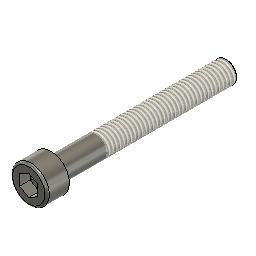
In-tube Belt Clamp (Autodesk Fusion 360 archive; units mm, degrees)
design "Hexagon Socket Head Cap Screw ANSI B18.3 - 10-32 UNF x 1 1/2 Steel Grade 2 Plain"
description: Hexagon Socket Head Cap Screw ANSI B18.3 - 10-32 UNF x 1 1/2
part number: HSHCS ANSI B18.3 - 10-32 UNF x 1 1/2 Steel Grade 2 Plain
Autodesk Fusion 360 part; units mm, degrees
sketch "Sketch1" plane through (0, 0, 0) normal (0, 1, 0) x (1, 0, 0)
  line L0 (-2.413, 0) -> (-2.413, 38.1)
  line L1 (-2.413, 38.1) -> (0, 38.1)
  line L2 (0, 38.1) -> (0, -4.826)
  line L3 (-2.413, 0) -> (-3.9624, 0)
  line L4 (-3.9624, 0) -> (-3.9624, -4.826)
  line L5 (-3.9624, -4.826) -> (0, -4.826)
  dimension "d107" = 4.826
  dimension "d108" = 38.1
  dimension "d114" = 7.9248
  dimension "d115" = 4.826
  constraint perpendicular L0 L1
  constraint collinear origin L1.end L2.end
  constraint perpendicular L0 L3
  constraint coincident origin L3
  constraint vertical L2
  constraint coincident L2 L5.end
  constraint perpendicular L2 L5
  measures "d107" distance of L3.end L5
  measures "d108" distance of origin L1
revolve "Revolve1" add sketch "Sketch1" angle 360 about axis through (0, 0, -38.1) along (0, 0, 1)
ref_plane "WorkPlane1" through (0, 0, 4.826) normal (0, 0, 1) x (1, 0, 0)
sketch "Sketch6" plane through (0, 0, 4.826) normal (0, 0, 1) x (1, 0, 0)
  line L0 (-1.9812, 1.1438) -> (-1.9812, -1.1438)
  line L1 (-1.9812, -1.1438) -> (0, -2.2877)
  line L2 (0, -2.2877) -> (1.9812, -1.1438)
  line L3 (1.9812, -1.1438) -> (1.9812, 1.1438)
  line L4 (1.9812, 1.1438) -> (0, 2.2877)
  line L5 (0, 2.2877) -> (-1.9812, 1.1438)
  dimension "d116" = 3.9624
  constraint vertical L3
  measures "d116" distance of L0 L3
extrude "Extrude1" cut sketch "Sketch6" against normal blind 2.286
extrude "Extrude2" cut 1 faces at (-0.6604, 0.3813, 2.54) along direction (0, 0, -1) blind 2.286 draft -85
thread "Thread3" "ANSI Unified Screw Threads 0.19(#10) 10-32 UNF 10-32 UNF 2A" major diameter 4.7269 minor diameter 3.8583 pitch 0.7937 angle 60 resizes the face on face at (-2.401, 0.2403, -25.4) from (0, 0, -9.652) to (0, 0, -38.1)
fillet "Fillet4" radius 0.4826 1 edges at (-3.6943, 1.4329, 4.826)
sketch "Sketch7" plane through (0, 0, 0) normal (0, 1, 0) x (1, 0, 0)
  line L0 (-2.4613, 38.1) -> (-2.4613, 37.6276)
  line L1 (-2.4613, 37.6276) -> (-1.9406, 38.1)
  line L2 (0, 38.1) -> (0, -4.826)
  line L3 (-2.4613, 38.1) -> (0, 38.1)
  dimension "d103" = 2.4613
  dimension "d110" = 1.9406
  dimension "d111" = 0.4724
  constraint coincident L2.start L3.end
  constraint perpendicular L2 L3
  constraint coincident L1.end L3
  constraint perpendicular L0 L3
  measures "d103" distance of origin L0
  measures "d110" distance of L1.end L2
  measures "d111" distance of L0.end L3
revolve "Revolve3" cut sketch "Sketch7" angle 360 about axis through (0, 0, 1.75) along (0, 0, 1)
equation "d31 = -adsk_phildepth"
equation "d71 = adsk_headh"
equation "d76 = -adsk_phildepth"
equation "adsk_nomlen = 1.50 in"
equation "adsk_headh = 0.19 in"
equation "adsk_headdia = 0.312 in"
equation "adsk_nomdia = 0.19 in"
equation "adsk_philwidth = 0.156 in"
equation "adsk_phildepth = 0.09 in"
equation "adsk_thrlen = 1.12 in"
equation "d93 = adsk_nomdia * 0.1"
equation "adsk_startlen = 0.0186 in"
equation "adsk_endpointdia = 0.1528 in"
equation "d103 = adsk_nomdia * 0.51"
equation "d107 = adsk_headh"
equation "d108 = adsk_nomlen"
equation "d110 = adsk_endpointdia / 2"
equation "d111 = adsk_startlen"
equation "d113 = min(adsk_thrlen; adsk_nomlen - 0.001 mm)"
equation "d114 = adsk_headdia"
equation "d115 = adsk_nomdia"
equation "d116 = adsk_philwidth"

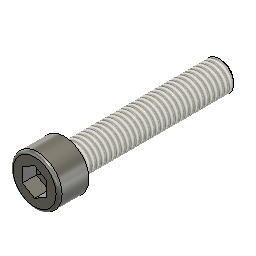
design "Hexagon Socket Head Cap Screw ANSI B18.3 - 10-32 UNF x 1 Steel Grade 2 Plain"
description: Hexagon Socket Head Cap Screw ANSI B18.3 - 10-32 UNF x 1
part number: HSHCS ANSI B18.3 - 10-32 UNF x 1 Steel Grade 2 Plain
Autodesk Fusion 360 part; units mm, degrees
sketch "Sketch1" plane through (0, 0, 0) normal (0, 1, 0) x (1, 0, 0)
  line L0 (-2.413, 0) -> (-2.413, 25.4)
  line L1 (-2.413, 25.4) -> (0, 25.4)
  line L2 (0, 25.4) -> (0, -4.826)
  line L3 (-2.413, 0) -> (-3.9624, 0)
  line L4 (-3.9624, 0) -> (-3.9624, -4.826)
  line L5 (-3.9624, -4.826) -> (0, -4.826)
  dimension "d107" = 4.826
  dimension "d108" = 25.4
  dimension "d114" = 7.9248
  dimension "d115" = 4.826
  constraint perpendicular L0 L1
  constraint collinear origin L1.end L2.end
  constraint perpendicular L0 L3
  constraint coincident origin L3
  constraint vertical L2
  constraint coincident L2 L5.end
  constraint perpendicular L2 L5
  measures "d107" distance of L3.end L5
  measures "d108" distance of origin L1
revolve "Revolve1" add sketch "Sketch1" angle 360 about axis through (0, 0, -25.4) along (0, 0, 1)
ref_plane "WorkPlane1" through (0, 0, 4.826) normal (0, 0, 1) x (1, 0, 0)
sketch "Sketch6" plane through (0, 0, 4.826) normal (0, 0, 1) x (1, 0, 0)
  line L0 (-1.9812, 1.1438) -> (-1.9812, -1.1438)
  line L1 (-1.9812, -1.1438) -> (0, -2.2877)
  line L2 (0, -2.2877) -> (1.9812, -1.1438)
  line L3 (1.9812, -1.1438) -> (1.9812, 1.1438)
  line L4 (1.9812, 1.1438) -> (0, 2.2877)
  line L5 (0, 2.2877) -> (-1.9812, 1.1438)
  dimension "d116" = 3.9624
  constraint vertical L3
  measures "d116" distance of L0 L3
extrude "Extrude1" cut sketch "Sketch6" against normal blind 2.286
extrude "Extrude2" cut 1 faces at (-0.6604, 0.3813, 2.54) along direction (0, 0, -1) blind 2.286 draft -85
thread "Thread3" "ANSI Unified Screw Threads 0.19(#10) 10-32 UNF 10-32 UNF 2A" major diameter 4.7269 minor diameter 3.8583 pitch 0.7937 angle 60 resizes the face on face at (-2.401, 0.2403, -16.9333) from (0, 0, -1.191) to (0, 0, -25.4)
fillet "Fillet4" radius 0.4826 1 edges at (-3.6943, 1.4329, 4.826)
sketch "Sketch7" plane through (0, 0, 0) normal (0, 1, 0) x (1, 0, 0)
  line L0 (-2.4613, 25.4) -> (-2.4613, 24.9276)
  line L1 (-2.4613, 24.9276) -> (-1.9406, 25.4)
  line L2 (0, 25.4) -> (0, -4.826)
  line L3 (-2.4613, 25.4) -> (0, 25.4)
  dimension "d103" = 2.4613
  dimension "d110" = 1.9406
  dimension "d111" = 0.4724
  constraint coincident L2.start L3.end
  constraint perpendicular L2 L3
  constraint coincident L1.end L3
  constraint perpendicular L0 L3
  measures "d103" distance of origin L0
  measures "d110" distance of L1.end L2
  measures "d111" distance of L0.end L3
revolve "Revolve3" cut sketch "Sketch7" angle 360 about axis through (0, 0, 1.75) along (0, 0, 1)
equation "d31 = -adsk_phildepth"
equation "d71 = adsk_headh"
equation "d76 = -adsk_phildepth"
equation "adsk_nomlen = 1.00 in"
equation "adsk_headh = 0.19 in"
equation "adsk_headdia = 0.312 in"
equation "adsk_nomdia = 0.19 in"
equation "adsk_philwidth = 0.156 in"
equation "adsk_phildepth = 0.09 in"
equation "adsk_thrlen = 0.9531121 in"
equation "d93 = adsk_nomdia * 0.1"
equation "adsk_startlen = 0.0186 in"
equation "adsk_endpointdia = 0.1528 in"
equation "d103 = adsk_nomdia * 0.51"
equation "d107 = adsk_headh"
equation "d108 = adsk_nomlen"
equation "d110 = adsk_endpointdia / 2"
equation "d111 = adsk_startlen"
equation "d113 = min(adsk_thrlen; adsk_nomlen - 0.001 mm)"
equation "d114 = adsk_headdia"
equation "d115 = adsk_nomdia"
equation "d116 = adsk_philwidth"

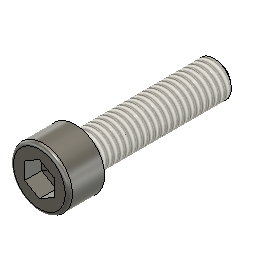
design "Hexagon Socket Head Cap Screw ANSI B18.3 - 10-32 UNF x 3/4 Steel Grade 2 Plain"
description: Hexagon Socket Head Cap Screw ANSI B18.3 - 10-32 UNF x 3/4
part number: HSHCS ANSI B18.3 - 10-32 UNF x 3/4 Steel Grade 2 Plain
Autodesk Fusion 360 part; units mm, degrees
sketch "Sketch1" plane through (0, 0, 0) normal (0, 1, 0) x (1, 0, 0)
  line L0 (-2.413, 0) -> (-2.413, 19.05)
  line L1 (-2.413, 19.05) -> (0, 19.05)
  line L2 (0, 19.05) -> (0, -4.826)
  line L3 (-2.413, 0) -> (-3.9624, 0)
  line L4 (-3.9624, 0) -> (-3.9624, -4.826)
  line L5 (-3.9624, -4.826) -> (0, -4.826)
  dimension "d107" = 4.826
  dimension "d108" = 19.05
  dimension "d114" = 7.9248
  dimension "d115" = 4.826
  constraint perpendicular L0 L1
  constraint collinear origin L1.end L2.end
  constraint perpendicular L0 L3
  constraint coincident origin L3
  constraint vertical L2
  constraint coincident L2 L5.end
  constraint perpendicular L2 L5
  measures "d107" distance of L3.end L5
  measures "d108" distance of origin L1
revolve "Revolve1" add sketch "Sketch1" angle 360 about axis through (0, 0, -19.05) along (0, 0, 1)
ref_plane "WorkPlane1" through (0, 0, 4.826) normal (0, 0, 1) x (1, 0, 0)
sketch "Sketch6" plane through (0, 0, 4.826) normal (0, 0, 1) x (1, 0, 0)
  line L0 (-1.9812, 1.1438) -> (-1.9812, -1.1438)
  line L1 (-1.9812, -1.1438) -> (0, -2.2877)
  line L2 (0, -2.2877) -> (1.9812, -1.1438)
  line L3 (1.9812, -1.1438) -> (1.9812, 1.1438)
  line L4 (1.9812, 1.1438) -> (0, 2.2877)
  line L5 (0, 2.2877) -> (-1.9812, 1.1438)
  dimension "d116" = 3.9624
  constraint vertical L3
  measures "d116" distance of L0 L3
extrude "Extrude1" cut sketch "Sketch6" against normal blind 2.286
extrude "Extrude2" cut 1 faces at (-0.6604, 0.3813, 2.54) along direction (0, 0, -1) blind 2.286 draft -85
thread "Thread3" "ANSI Unified Screw Threads 0.19(#10) 10-32 UNF 10-32 UNF 2A" major diameter 4.7269 minor diameter 3.8583 pitch 0.7937 angle 60 resizes the face on face at (-2.401, 0.2403, -12.7) from (0, 0, -1.191) to (0, 0, -19.05)
fillet "Fillet4" radius 0.4826 1 edges at (-3.6943, 1.4329, 4.826)
sketch "Sketch7" plane through (0, 0, 0) normal (0, 1, 0) x (1, 0, 0)
  line L0 (-2.4613, 19.05) -> (-2.4613, 18.5776)
  line L1 (-2.4613, 18.5776) -> (-1.9406, 19.05)
  line L2 (0, 19.05) -> (0, -4.826)
  line L3 (-2.4613, 19.05) -> (0, 19.05)
  dimension "d103" = 2.4613
  dimension "d110" = 1.9406
  dimension "d111" = 0.4724
  constraint coincident L2.start L3.end
  constraint perpendicular L2 L3
  constraint coincident L1.end L3
  constraint perpendicular L0 L3
  measures "d103" distance of origin L0
  measures "d110" distance of L1.end L2
  measures "d111" distance of L0.end L3
revolve "Revolve3" cut sketch "Sketch7" angle 360 about axis through (0, 0, 1.75) along (0, 0, 1)
equation "d31 = -adsk_phildepth"
equation "d71 = adsk_headh"
equation "d76 = -adsk_phildepth"
equation "adsk_nomlen = 0.75 in"
equation "adsk_headh = 0.19 in"
equation "adsk_headdia = 0.312 in"
equation "adsk_nomdia = 0.19 in"
equation "adsk_philwidth = 0.156 in"
equation "adsk_phildepth = 0.09 in"
equation "adsk_thrlen = 0.7031121 in"
equation "d93 = adsk_nomdia * 0.1"
equation "adsk_startlen = 0.0186 in"
equation "adsk_endpointdia = 0.1528 in"
equation "d103 = adsk_nomdia * 0.51"
equation "d107 = adsk_headh"
equation "d108 = adsk_nomlen"
equation "d110 = adsk_endpointdia / 2"
equation "d111 = adsk_startlen"
equation "d113 = min(adsk_thrlen; adsk_nomlen - 0.001 mm)"
equation "d114 = adsk_headdia"
equation "d115 = adsk_nomdia"
equation "d116 = adsk_philwidth"

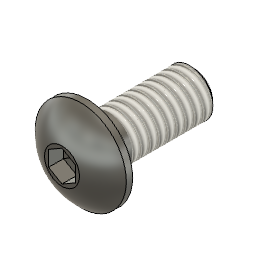
design "Hexagon Socket Button Head Cap Screw ANSI B18.3 - #4-48 x 1/4 Steel Grade 2 Plain"
description: Hexagon Socket Button Head Cap Screw ANSI B18.3 - #4-48 x 1/4
part number: HSBHCS ANSI B18.3 - #4-48 x 1/4 Steel Grade 2 Plain
Autodesk Fusion 360 part; units mm, degrees
sketch "Sketch1" plane through (0, 0, 0) normal (0, 1, 0) x (1, 0, 0)
  line L0 (-1.4224, 0) -> (-1.4224, 6.35)
  line L1 (-1.4224, 6.35) -> (0, 6.35)
  line L2 (0, 6.35) -> (0, -1.4986)
  line L3 (-1.4224, 0) -> (-2.7051, 0)
  line L4 (0, -1.4986) -> (-1.0401, -1.4986)
  line L5 (-2.7051, 0) -> (-2.7051, -0.381)
  arc A0 (-2.7051, -0.381) -> (-1.0401, -1.4986) centre (0, 1.85) ccw
  dimension "d9" = 2.8448
  dimension "d66" = 5.4102
  dimension "d129" = 2.0803
  dimension "d130" = 6.35
  dimension "d131" = 1.4986
  dimension "d132" = 0.381
  constraint perpendicular L0 L1
  constraint perpendicular L0 L3
  constraint coincident origin L3
  constraint vertical L0
  constraint vertical L2
  constraint perpendicular L2 L4
  constraint coincident origin L2
  constraint perpendicular L3 L5
  constraint coincident L2 A0.centre
  measures "d130" distance of origin L1
  measures "d131" distance of L3 L4.end
  measures "d132" distance of L3 L5.end
revolve "Revolve1" add sketch "Sketch1" angle 360 about axis through (0, 0, -6.35) along (0, 0, 1)
ref_plane "WorkPlane1" through (0, 0, 1.4986) normal (0, 0, 1) x (1, 0, 0)
sketch "Sketch6" plane through (0, 0, 1.4986) normal (0, 0, 1) x (1, 0, 0)
  line L0 (0, -0.9239) -> (0.8001, -0.4619)
  line L1 (0.8001, -0.4619) -> (0.8001, 0.4619)
  line L2 (0.8001, 0.4619) -> (0, 0.9239)
  line L3 (0, 0.9239) -> (-0.8001, 0.4619)
  line L4 (-0.8001, 0.4619) -> (-0.8001, -0.4619)
  line L5 (-0.8001, -0.4619) -> (0, -0.9239)
  dimension "d143" = 1.6002
  constraint vertical L1
  measures "d143" distance of L1 L4
extrude "Extrude1" cut sketch "Sketch6" against normal blind 0.889
extrude "Extrude2" cut 1 faces at (0, -0.308, 0.6096) along direction (0, 0, -1) blind 0.889 draft -85
fillet "Fillet5" radius 0.1422 1 edges at (-1.3261, 0.5144, 0)
thread "Thread5" "ANSI Unified Screw Threads 0.112(#4) 4-48 UNF 4-48 UNF 2A" major diameter 2.7711 minor diameter 2.1946 pitch 0.5292 angle 60 resizes the face on face at (-1.4206, 0.0709, -2.2115) from (0, 0, -1.2702) to (0, 0, -6.35)
sketch "Sketch7" plane through (0, 0, 0) normal (0, 1, 0) x (1, 0, 0)
  line L0 (-1.4508, 6.35) -> (-1.4508, 6.0338)
  line L1 (-1.4508, 6.0338) -> (-1.1062, 6.35)
  line L2 (0, 6.35) -> (0, -1.4986)
  line L3 (-1.4508, 6.35) -> (0, 6.35)
  dimension "d134" = 0.3162
  dimension "d135" = 1.1062
  dimension "d136" = 1.4508
  constraint coincident L2.start L3.end
  constraint perpendicular L2 L3
  constraint coincident L1.end L3
  constraint perpendicular L0 L3
  measures "d134" distance of L0.end L3
  measures "d135" distance of L1.end L2
  measures "d136" distance of L0.start L2
revolve "Revolve3" cut sketch "Sketch7" angle 360 about axis through (0, 0, 1.75) along (0, 0, 1)
equation "d9 = adsk_nomdia"
equation "d31 = -adsk_phildepth"
equation "d66 = adsk_headdia"
equation "d71 = adsk_headh"
equation "d76 = -adsk_phildepth"
equation "adsk_nomlen = 0.25 in"
equation "adsk_headh = 0.059 in"
equation "adsk_headdia = 0.213 in"
equation "adsk_nomdia = 0.112 in"
equation "adsk_philwidth = 0.063 in"
equation "adsk_phildepth = 0.035 in"
equation "adsk_thrlen = 0.1999921 in"
equation "adsk_endpointdia = 0.0871 in"
equation "adsk_startlen = 0.01245 in"
equation "adsk_midfillet = adsk_nomdia * 0.05"
equation "d114 = adsk_midfillet"
equation "adsk_baseh = 0.015 in"
equation "d129 = adsk_philwidth * 1.3"
equation "d130 = adsk_nomlen"
equation "d131 = adsk_headh"
equation "d132 = adsk_baseh"
equation "d134 = adsk_startlen"
equation "d135 = adsk_endpointdia / 2"
equation "d136 = adsk_nomdia * 0.51"
equation "d142 = min(adsk_thrlen; adsk_nomlen - adsk_midfillet - 0.001 mm)"
equation "d143 = adsk_philwidth"
